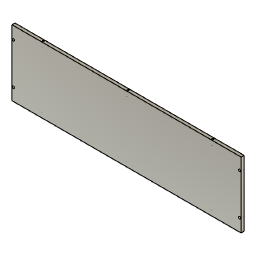
wheel body v234 (Autodesk Fusion 360 archive; units mm, degrees)
design "side_cover_front_wall"
Autodesk Fusion 360 part; units mm, degrees
note: some values were not read from the file. Chosen so that the rebuilt part matches the saved one: which face or edge a step refers to; how an offset face is resized; which pieces of a blend or face edit are solid.
sketch "Sketch1" plane through (0, 0, 0) normal (0, 1, 0) x (1, 0, 0)
  line L0 (0, 0) -> (470, 0)
  line L1 (470, 0) -> (470, -137.719)
  line L2 (470, -137.719) -> (0, -137.719)
  line L3 (0, -137.719) -> (0, 0)
  dimension "d1" = 470
  dimension "d2" = 137.719
  constraint horizontal L0
  constraint vertical L1
  constraint horizontal L2
  constraint vertical L3
  constraint coincident L0.start L3.end
  measures "d1" distance of L0.start L0.end
  measures "d2" distance of L0.start L2.end
extrude "Extrude1" add sketch "Sketch1" along normal blind 10
sketch "Sketch2" plane through (0, 0, 0) normal (0, -1, 0) x (1, 0, 0)
  line L0 (470, 137.719) -> (0, 137.719)
  line L1 (0, 137.719) -> (0, 0)
  line L2 (0, 0) -> (470, 0)
  line L3 (470, 0) -> (470, 137.719)
  line L4 (470, 0) -> (465, 0)
  line L5 (465, 0) -> (465, 25)
  line L6 (465, 25) -> (470, 25)
  line L7 (470, 25) -> (470, 0)
  line L8 (470, 137.719) -> (465, 137.719)
  line L9 (465, 137.719) -> (465, 112.719)
  line L10 (465, 112.719) -> (470, 112.719)
  line L11 (470, 112.719) -> (470, 137.719)
  line L12 (0, 137.719) -> (5, 137.719)
  line L13 (5, 137.719) -> (5, 112.719)
  line L14 (5, 112.719) -> (0, 112.719)
  line L15 (0, 112.719) -> (0, 137.719)
  line L16 (0, 0) -> (5, 0)
  line L17 (5, 0) -> (5, 25)
  line L18 (5, 25) -> (0, 25)
  line L19 (0, 25) -> (0, 0)
  dimension "d5" = 5
  dimension "d6" = 25
  dimension "d7" = 25
  dimension "d8" = 5
  dimension "d9" = 25
  dimension "d10" = 5
  dimension "d11" = 25
  constraint horizontal L4
  constraint vertical L5
  constraint horizontal L6
  constraint vertical L7
  constraint coincident L2.end L3.start
  constraint horizontal L8
  constraint vertical L9
  constraint horizontal L10
  constraint vertical L11
  constraint coincident L0.start L3.end
  constraint horizontal L12
  constraint vertical L13
  constraint horizontal L14
  constraint vertical L15
  constraint coincident L0.end L1.start
  constraint horizontal L16
  constraint vertical L17
  constraint horizontal L18
  constraint vertical L19
  constraint coincident L1.end L2.start
  measures "d5" distance of L2.end L4.end
  measures "d6" distance of L2.end L6.end
  measures "d7" distance of L0.start L10.end
  measures "d8" distance of L0.end L12.end
  measures "d9" distance of L0.end L14.end
  measures "d10" distance of L1.end L16.end
  measures "d11" distance of L1.end L18.end
sketch "Sketch3" plane through (0, 0, 137.719) normal (0, 0, 1) x (-1, 0, 0)
  line L0 (0, 0) -> (-470, 0)
  line L1 (-470, 0) -> (-470, -10)
  line L2 (-470, -10) -> (0, -10)
  line L3 (0, -10) -> (0, 0)
  line L4 (0, -5) -> (-60, -5)
  line L5 (-470, -5) -> (-410, -5)
  line L6 (-60, -5) -> (-235, -5)
  dimension "d15" = 60
  dimension "d16" = 60
  dimension "d17" = 175
  constraint midpoint L3 L4.start
  constraint perpendicular L3 L4
  constraint midpoint L1 L5.start
  constraint perpendicular L1 L5
  constraint parallel L5 L6
  measures "d15" distance of L4.start L4.end
  measures "d16" distance of L5.start L5.end
  measures "d17" distance of L4.end L6.end
extrude "Extrude2" cut 1 faces at (313.3333, 10, 91.8127) along direction (0, -1, 0) blind 4
extrude "Extrude3" cut 1 faces at (470, 2, 45.9063) along direction (-1, 0, 0) blind 4
extrude "Extrude4" cut 1 faces at (0, 2, 91.8127) along direction (1, 0, 0) blind 4
sketch "Sketch4" plane through (4, 0, 0) normal (-1, 0, 0) x (0, -1, 0)
  line L0 (-6, 137.719) -> (-6, 0)
  line L1 (-6, 0) -> (0, 0)
  line L2 (0, 0) -> (0, 137.719)
  line L3 (0, 137.719) -> (-6, 137.719)
  line L4 (-3, 0) -> (-3, 25)
  line L5 (-3, 137.719) -> (-3, 112.719)
  dimension "d27" = 25
  dimension "d28" = 25
  constraint midpoint L1 L4.start
  constraint perpendicular L1 L4
  constraint midpoint L3 L5.start
  constraint perpendicular L3 L5
  measures "d27" distance of L4.start L4.end
  measures "d28" distance of L5.start L5.end
hole "Hole3" at (4, 3, 112.719) at (4, 3, 25) direction (1, 0, 0) diameter 3.332 depth 10 tip angle 180
thread "Thread3" "ISO Metric profile 4.0 M4x0.5 6H" major diameter 4.0861 minor diameter 3.5287 pitch 0.5 angle 60 resizes the face on face at (7.3333, 1.3345, 112.6775) on face at (7.3333, 3.083, 26.6639)
sketch "Sketch5" plane through (466, 0, 0) normal (1, 0, 0) x (0, 1, 0)
  line L0 (6, 0) -> (6, 137.719)
  line L1 (6, 137.719) -> (0, 137.719)
  line L2 (0, 137.719) -> (0, 0)
  line L3 (0, 0) -> (6, 0)
  line L4 (3, 0) -> (3, 25)
  line L5 (3, 137.719) -> (3, 112.719)
  dimension "d32" = 25
  dimension "d33" = 25
  constraint midpoint L3 L4.start
  constraint perpendicular L3 L4
  constraint midpoint L1 L5.start
  constraint perpendicular L1 L5
  measures "d32" distance of L4.start L4.end
  measures "d33" distance of L5.start L5.end
sketch "Sketch6" plane through (0, 0, 137.719) normal (0, 0, 1) x (-1, 0, 0)
  line L0 (-4, -6) -> (-4, 0)
  line L1 (-4, 0) -> (-466, 0)
  line L2 (-466, 0) -> (-466, -6)
  line L3 (-466, -6) -> (-4, -6)
  line L4 (-4, -3) -> (-64, -3)
  line L5 (-466, -3) -> (-406, -3)
  line L6 (-406, -3) -> (-235, -3)
  dimension "d37" = 60
  dimension "d38" = 60
  dimension "d39" = 171
  constraint midpoint L0 L4.start
  constraint perpendicular L0 L4
  constraint midpoint L2 L5.start
  constraint perpendicular L2 L5
  constraint parallel L3 L6
  measures "d37" distance of L4.start L4.end
  measures "d38" distance of L5.start L5.end
  measures "d39" distance of L5.end L6.end
hole "Hole5" at (64, 3, 137.719) at (235, 3, 137.719) at (406, 3, 137.719) direction (0, 0, -1) diameter 3.529 depth 10 tip angle 180
thread "Thread5" "ISO Metric profile 4.0 M4x0.5 6H"
delete_face "DeleteFace1" 1 faces at (10.6667, 1.2362, 112.763)
delete_face "DeleteFace2" 1 faces at (10.6667, 3.1757, 26.7556)
sketch "Sketch7" plane through (0, 6, 0) normal (0, 1, 0) x (-1, 0, 0)
  line L0 (-4, 0) -> (-4, 137.719)
  line L1 (-4, 137.719) -> (-466, 137.719)
  line L2 (-466, 137.719) -> (-466, 0)
  line L3 (-466, 0) -> (-4, 0)
  line L4 (-466, 137.719) -> (-463, 137.719)
  line L5 (-463, 137.719) -> (-463, 112.719)
  line L6 (-463, 112.719) -> (-466, 112.719)
  line L7 (-466, 112.719) -> (-466, 137.719)
  dimension "d43" = 3
  dimension "d44" = 25
  constraint horizontal L4
  constraint vertical L5
  constraint horizontal L6
  constraint vertical L7
  constraint coincident L1.end L2.start
  measures "d43" distance of L1.end L4.end
  measures "d44" distance of L1.end L6.end
hole "Hole6" at (463, 6, 112.719) direction (0, -1, 0) diameter 4.5 depth 80 tip angle 180
sketch "Sketch8" plane through (0, 6, 0) normal (0, 1, 0) x (-1, 0, 0)
  circle A0 centre (-463, 112.719) radius 2.25
  line L0 (-4, 0) -> (-4, 137.719)
  line L1 (-4, 137.719) -> (-466, 137.719)
  line L2 (-466, 137.719) -> (-466, 0)
  line L3 (-466, 0) -> (-4, 0)
  line L4 (-466, 0) -> (-463, 0)
  line L5 (-463, 0) -> (-463, 25)
  line L6 (-463, 25) -> (-466, 25)
  line L7 (-466, 25) -> (-466, 0)
  line L8 (-4, 137.719) -> (-7, 137.719)
  line L9 (-7, 137.719) -> (-7, 112.719)
  line L10 (-7, 112.719) -> (-4, 112.719)
  line L11 (-4, 112.719) -> (-4, 137.719)
  line L12 (-4, 0) -> (-7, 0)
  line L13 (-7, 0) -> (-7, 25)
  line L14 (-7, 25) -> (-4, 25)
  line L15 (-4, 25) -> (-4, 0)
  dimension "d48" = 3
  dimension "d49" = 25
  dimension "d50" = 3
  dimension "d51" = 25
  dimension "d52" = 3
  dimension "d53" = 25
  constraint horizontal L4
  constraint vertical L5
  constraint horizontal L6
  constraint vertical L7
  constraint coincident L2.end L3.start
  constraint horizontal L8
  constraint vertical L9
  constraint horizontal L10
  constraint vertical L11
  constraint coincident L0.end L1.start
  constraint horizontal L12
  constraint vertical L13
  constraint horizontal L14
  constraint vertical L15
  constraint coincident L0.start L3.end
  measures "d48" distance of L2.end L4.end
  measures "d49" distance of L2.end L6.end
  measures "d50" distance of L0.end L8.end
  measures "d51" distance of L0.end L10.end
  measures "d52" distance of L0.start L12.end
  measures "d53" distance of L0.start L14.end
hole "Hole7" at (7, 6, 112.719) at (7, 6, 25) at (463, 6, 25) direction (0, -1, 0) diameter 4.5 depth 80 tip angle 180
extrude "Extrude5" cut 1 faces at (158, 2, 0) along direction (0, 0, 1) blind 4
extrude "Extrude6" cut 1 faces at (158, 2, 4) along direction (0, 0, 1) blind 1
sketch "Sketch9" plane through (0, 0, 5) normal (0, 0, -1) x (1, 0, 0)
  line L0 (4, 0) -> (4, -6)
  line L1 (4, -6) -> (466, -6)
  line L2 (466, -6) -> (466, 0)
  line L3 (466, 0) -> (4, 0)
  line L4 (466, -3) -> (406, -3)
  line L5 (406, -3) -> (235, -3)
  line L6 (235, -3) -> (64, -3)
  dimension "d61" = 60
  dimension "d62" = 171
  constraint midpoint L2 L4.start
  constraint perpendicular L2 L4
  constraint parallel L3 L5
  constraint perpendicular L0 L6
  measures "d61" distance of L4.start L4.end
  measures "d62" distance of L5.end L6.end
hole "Hole8" at (64, 3, 5) at (235, 3, 5) at (406, 3, 5) direction (0, 0, 1) diameter 3.529 depth 10 tip angle 180
thread "Thread6" "ISO Metric profile 4.0 M4x0.5 6H"
extrude "Extrude7" add 1 faces at (466, 2, 49.2397) along direction (1, 0, 0) blind 0.502
delete_face "DeleteFace3" 1 faces at (462.4448, 4, 114.8994)
delete_face "DeleteFace4" 1 faces at (462.4448, 4, 27.1804)
sketch "Sketch10" plane through (0, 0, 0) normal (0, -1, 0) x (1, 0, 0)
  circle A0 centre (7, 112.719) radius 2.25
  circle A1 centre (7, 25) radius 2.25
  line L0 (4, 5) -> (466.502, 5)
  line L1 (466.502, 5) -> (466.502, 137.719)
  line L2 (466.502, 137.719) -> (4, 137.719)
  line L3 (4, 137.719) -> (4, 5)
  line L4 (466.502, 137.719) -> (463.502, 137.719)
  line L5 (463.502, 137.719) -> (463.502, 112.719)
  line L6 (463.502, 112.719) -> (466.502, 112.719)
  line L7 (466.502, 112.719) -> (466.502, 137.719)
  line L8 (466.502, 5) -> (463.502, 5)
  line L9 (463.502, 5) -> (463.502, 30)
  line L10 (463.502, 30) -> (466.502, 30)
  line L11 (466.502, 30) -> (466.502, 5)
  dimension "d68" = 3
  dimension "d69" = 25
  dimension "d70" = 3
  dimension "d71" = 25
  constraint horizontal L4
  constraint vertical L5
  constraint horizontal L6
  constraint vertical L7
  constraint coincident L1.end L2.start
  constraint horizontal L8
  constraint vertical L9
  constraint horizontal L10
  constraint vertical L11
  constraint coincident L0.end L1.start
  measures "d68" distance of L1.end L4.end
  measures "d69" distance of L1.end L6.end
  measures "d70" distance of L0.end L8.end
  measures "d71" distance of L0.end L10.end
hole "Hole9" at (463.502, 0, 30) at (463.502, 0, 112.719) direction (0, 1, 0) diameter 4.5 depth 40 tip angle 180
sketch "Sketch11" plane through (0, 0, 0) normal (0, -1, 0) x (1, 0, 0)
  circle A0 centre (463.502, 30) radius 2.25
  circle A1 centre (463.502, 112.719) radius 2.25
  circle A2 centre (7, 112.719) radius 2.25
  circle A3 centre (7, 25) radius 2.25
  line L0 (4, 5) -> (466.502, 5)
  line L1 (466.502, 5) -> (466.502, 137.719)
  line L2 (466.502, 137.719) -> (4, 137.719)
  line L3 (4, 137.719) -> (4, 5)
  line L4 (4, 5) -> (7, 5)
  line L5 (7, 5) -> (7, 30)
  line L6 (7, 30) -> (4, 30)
  line L7 (4, 30) -> (4, 5)
  dimension "d75" = 3
  dimension "d76" = 25
  constraint horizontal L4
  constraint vertical L5
  constraint horizontal L6
  constraint vertical L7
  constraint coincident L0.start L3.end
  measures "d75" distance of L0.start L4.end
  measures "d76" distance of L0.start L6.end
hole "Hole10" at (7, 0, 30) direction (0, 1, 0) diameter 4.5 depth 10 tip angle 180
delete_face "DeleteFace5" 1 faces at (7.224, 2, 27.2388)
delete_face "DeleteFace6" 2 faces at (404.8658, 4.3517, 134.3857) (405.4525, 2.6972, 127.719)
sketch "Sketch12" plane through (0, 0, 137.719) normal (0, 0, 1) x (-1, 0, 0)
  circle A0 centre (-235, -3) radius 1.7644
  circle A1 centre (-64, -3) radius 1.7644
  line L0 (-4, -6) -> (-4, 0)
  line L1 (-4, 0) -> (-466.502, 0)
  line L2 (-466.502, 0) -> (-466.502, -6)
  line L3 (-466.502, -6) -> (-4, -6)
  line L4 (-466.502, -3) -> (-406.502, -3)
  dimension "d80" = 60
  constraint midpoint L2 L4.start
  constraint perpendicular L2 L4
  measures "d80" distance of L4.start L4.end
hole "Hole11" at (406.502, 3, 137.719) direction (0, 0, -1) diameter 3.332 depth 10 tip angle 180
thread "Thread7" "ISO Metric profile 4.0 M4x0.5 6H" major diameter 4.0861 minor diameter 3.5287 pitch 0.5 angle 60 resizes the face on face at (406.6679, 4.6577, 134.3857)
delete_face "DeleteFace7" 1 faces at (235.9201, 4.5056, 134.3857)
sketch "Sketch13" plane through (0, 0, 137.719) normal (0, 0, 1) x (-1, 0, 0)
  circle A0 centre (-406.502, -3) radius 1.7644
  circle A1 centre (-64, -3) radius 1.7644
  line L0 (-4, -6) -> (-4, 0)
  line L1 (-4, 0) -> (-466.502, 0)
  line L2 (-466.502, 0) -> (-466.502, -6)
  line L3 (-466.502, -6) -> (-4, -6)
  line L4 (-64, -3) -> (-235.251, -3)
  dimension "d84" = 171.251
  constraint coincident A1.centre L4.start
  constraint parallel L1 L4
  measures "d84" distance of A1.centre L4.end
hole "Hole12" at (235.251, 3, 137.719) direction (0, 0, -1) diameter 3.332 depth 10 tip angle 180
thread "Thread8" "ISO Metric profile 4.0 M4x0.5 6H" major diameter 4.0861 minor diameter 3.5287 pitch 0.5 angle 60 resizes the face on face at (235.334, 1.3361, 134.3857)
delete_face "DeleteFace8" 1 faces at (404.9346, 4.4065, 8.3333)
sketch "Sketch14" plane through (0, 0, 5) normal (0, 0, -1) x (1, 0, 0)
  circle A0 centre (235, -3) radius 1.7644
  circle A1 centre (64, -3) radius 1.7644
  line L0 (4, 0) -> (4, -6)
  line L1 (4, -6) -> (466.502, -6)
  line L2 (466.502, -6) -> (466.502, 0)
  line L3 (466.502, 0) -> (4, 0)
  line L4 (466.502, -3) -> (406.502, -3)
  dimension "d88" = 60
  constraint midpoint L2 L4.start
  constraint perpendicular L2 L4
  measures "d88" distance of L4.start L4.end
hole "Hole13" at (406.502, 3, 5) direction (0, 0, 1) diameter 3.332 depth 10 tip angle 180
thread "Thread9" "ISO Metric profile 4.0 M4x0.5 6H" major diameter 4.0861 minor diameter 3.5287 pitch 0.5 angle 60 resizes the face on face at (406.585, 4.6639, 8.3333)
delete_face "DeleteFace9" 1 faces at (235.9201, 1.4944, 8.3333)
sketch "Sketch15" plane through (0, 0, 5) normal (0, 0, -1) x (1, 0, 0)
  circle A0 centre (406.502, -3) radius 1.7644
  circle A1 centre (64, -3) radius 1.7644
  line L0 (4, 0) -> (4, -6)
  line L1 (4, -6) -> (466.502, -6)
  line L2 (466.502, -6) -> (466.502, 0)
  line L3 (466.502, 0) -> (4, 0)
  line L4 (64, -3) -> (235.251, -3)
  dimension "d92" = 171.251
  constraint coincident A1.centre L4.start
  constraint parallel L3 L4
  measures "d92" distance of A1.centre L4.end
hole "Hole14" at (235.251, 3, 5) direction (0, 0, 1) diameter 3.529 depth 10 tip angle 180
thread "Thread10" "ISO Metric profile 4.0 M4x0.5 6H"
equation "d17 = ( 350.000 / 2 ) * 1 mm"
equation "d39 = ( 342.000 / 2 ) * 1 mm"
equation "d62 = 231.000 mm - 60 mm"
equation "d84 = ( 342.502 / 2 ) * 1 mm"
equation "d92 = ( 342.502 / 2 ) * 1 mm"

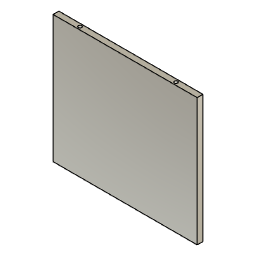
design "side_cover_side_wall"
Autodesk Fusion 360 part; units mm, degrees
sketch "Sketch1" plane through (0, 0, 0) normal (0, 0, 1) x (1, 0, 0)
  line L0 (0, 0) -> (150, 0)
  line L1 (150, 0) -> (150, 10)
  line L2 (150, 10) -> (0, 10)
  line L3 (0, 10) -> (0, 0)
  dimension "d1" = 150
  dimension "d2" = 10
  constraint horizontal L0
  constraint vertical L1
  constraint horizontal L2
  constraint vertical L3
  constraint coincident L0.start L3.end
  measures "d1" distance of L0.start L0.end
  measures "d2" distance of L0.start L2.end
extrude "Extrude1" add sketch "Sketch1" along normal blind 137.719
sketch "Sketch2" plane through (0, 0, 137.719) normal (0, 0, 1) x (-1, 0, 0)
  line L0 (0, -10) -> (0, 0)
  line L1 (0, 0) -> (-150, 0)
  line L2 (-150, 0) -> (-150, -10)
  line L3 (-150, -10) -> (0, -10)
  line L4 (0, -5) -> (-25, -5)
  line L5 (-150, -5) -> (-125, -5)
  dimension "d5" = 25
  dimension "d6" = 25
  constraint midpoint L0 L4.start
  constraint perpendicular L0 L4
  constraint midpoint L2 L5.start
  constraint perpendicular L2 L5
  measures "d5" distance of L4.start L4.end
  measures "d6" distance of L5.start L5.end
sketch "Sketch3" plane through (0, 0, 0) normal (-1, 0, 0) x (0, -1, 0)
  line L0 (-10, 0) -> (0, 0)
  line L1 (0, 0) -> (0, 137.719)
  line L2 (0, 137.719) -> (-10, 137.719)
  line L3 (-10, 137.719) -> (-10, 0)
  line L4 (-5, 0) -> (-5, 25)
  line L5 (-5, 137.719) -> (-5, 112.719)
  dimension "d10" = 25
  dimension "d11" = 25
  constraint parallel L3 L4
  constraint midpoint L2 L5.start
  constraint perpendicular L2 L5
  measures "d10" distance of L4.start L4.end
  measures "d11" distance of L5.start L5.end
extrude "Extrude2" cut 1 faces at (100, 10, 45.9063) along direction (0, -1, 0) blind 4
sketch "Sketch4" plane through (0, 0, 137.719) normal (0, 0, 1) x (-1, 0, 0)
  line L0 (-150, -6) -> (0, -6)
  line L1 (0, -6) -> (0, 0)
  line L2 (0, 0) -> (-150, 0)
  line L3 (-150, 0) -> (-150, -6)
  line L4 (0, -3) -> (-31, -3)
  line L5 (-150, -3) -> (-125, -3)
  dimension "d17" = 31
  dimension "d18" = 25
  constraint midpoint L1 L4.start
  constraint perpendicular L1 L4
  constraint midpoint L3 L5.start
  constraint perpendicular L3 L5
  measures "d17" distance of L4.start L4.end
  measures "d18" distance of L5.start L5.end
hole "Hole3" at (31, 3, 137.719) at (125, 3, 137.719) direction (0, 0, -1) diameter 3.529 depth 10 tip angle 180
thread "Thread3" "ISO Metric profile 4.0 M4x0.5 6H"
sketch "Sketch5" plane through (0, 0, 0) normal (-1, 0, 0) x (0, -1, 0)
  line L0 (-6, 137.719) -> (-6, 0)
  line L1 (-6, 0) -> (0, 0)
  line L2 (0, 0) -> (0, 137.719)
  line L3 (0, 137.719) -> (-6, 137.719)
  line L4 (-3, 137.719) -> (-3, 112.719)
  line L5 (-3, 0) -> (-3, 25)
  dimension "d22" = 25
  dimension "d23" = 25
  constraint midpoint L3 L4.start
  constraint perpendicular L3 L4
  constraint midpoint L1 L5.start
  constraint perpendicular L1 L5
  measures "d22" distance of L4.start L4.end
  measures "d23" distance of L5.start L5.end
hole "Hole4" at (0, 3, 112.719) at (0, 3, 25) direction (1, 0, 0) diameter 3.529 depth 10 tip angle 180
thread "Thread4" "ISO Metric profile 4.0 M4x0.5 6H"
delete_face "DeleteFace1" 1 faces at (31.088, 1.2377, 134.3857)
sketch "Sketch6" plane through (0, 0, 137.719) normal (0, 0, 1) x (-1, 0, 0)
  circle A0 centre (-125, -3) radius 1.7644
  line L0 (-150, -6) -> (0, -6)
  line L1 (0, -6) -> (0, 0)
  line L2 (0, 0) -> (-150, 0)
  line L3 (-150, 0) -> (-150, -6)
  line L4 (0, -3) -> (-25, -3)
  dimension "d27" = 25
  constraint midpoint L1 L4.start
  constraint perpendicular L1 L4
  measures "d27" distance of L4.start L4.end
hole "Hole5" at (25, 3, 137.719) direction (0, 0, -1) diameter 3.529 depth 10 tip angle 180
thread "Thread5" "ISO Metric profile 4.0 M4x0.5 6H"
extrude "Extrude3" cut 1 faces at (50, 4, 0) along direction (0, 0, 1) blind 4
extrude "Extrude4" cut 1 faces at (50, 4, 4) along direction (0, 0, 1) blind 1
sketch "Sketch7" plane through (0, 0, 5) normal (0, 0, -1) x (1, 0, 0)
  line L0 (0, -6) -> (150, -6)
  line L1 (150, -6) -> (150, 0)
  line L2 (150, 0) -> (0, 0)
  line L3 (0, 0) -> (0, -6)
  line L4 (0, -3) -> (25, -3)
  line L5 (150, -3) -> (125, -3)
  dimension "d35" = 25
  dimension "d36" = 25
  constraint midpoint L3 L4.start
  constraint perpendicular L3 L4
  constraint midpoint L1 L5.start
  constraint perpendicular L1 L5
  measures "d35" distance of L4.start L4.end
  measures "d36" distance of L5.start L5.end
hole "Hole6" at (25, 3, 5) at (125, 3, 5) direction (0, 0, 1) diameter 3.332 depth 10 tip angle 180
thread "Thread6" "ISO Metric profile 4.0 M4x0.5 6H" major diameter 4.0861 minor diameter 3.5287 pitch 0.5 angle 60 resizes the face on face at (25.083, 4.6639, 8.3333) on face at (126.0709, 1.7238, 8.3333)
sketch "Sketch8" plane through (0, 0, 0) normal (-1, 0, 0) x (0, -1, 0)
  circle A0 centre (-3, 112.719) radius 1.7644
  circle A1 centre (-3, 25) radius 1.7644
  line L0 (-6, 5) -> (0, 5)
  line L1 (0, 5) -> (0, 137.719)
  line L2 (0, 137.719) -> (-6, 137.719)
  line L3 (-6, 137.719) -> (-6, 5)
  line L4 (-3, 5) -> (-3, 30)
  dimension "d40" = 25
  constraint midpoint L0 L4.start
  constraint perpendicular L0 L4
  measures "d40" distance of L4.start L4.end
hole "Hole7" at (0, 3, 30) direction (1, 0, 0) diameter 3.332 depth 10 tip angle 180
thread "Thread7" "ISO Metric profile 4.0 M4x0.5 6H" major diameter 4.0861 minor diameter 3.5287 pitch 0.5 angle 60 resizes the face on face at (3.3333, 3.083, 31.6639)
delete_face "DeleteFace2" 2 faces at (6.6667, 3.1757, 26.7557) (10, 3.2552, 25.5942)
